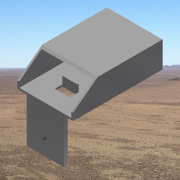
# Autodesk Inventor part: 2p1hh
Saved by Autodesk Inventor 2014 SP1 (Build 180222100, 222)
## iProperties
Company: HERA Project
Created: 2013-12-03
Part Number: 2p1hh
Material: Steel, Galvanized
Document SubType Name: Modeling
Designer: David DeBoer
Mass: 1619.54 g
Surface Area: 865.184 cm^2
Volume: 206.311 cm^3
Density: 7.85 g/cm^3
Description: end horizontal holder
Appearance: Galvanized
Author: David DeBoer
Autodesk Inventor part; units mm, degrees
ref_plane "YZ Plane" through (0, 0, 0) normal (1, 0, 0) x (0, 1, 0)
ref_plane "XZ Plane" through (0, 0, 0) normal (0, 1, 0) x (-1, 0, 0)
ref_plane "XY Plane" through (0, 0, 0) normal (0, 0, 1) x (1, 0, 0)
sketch "Sketch1" plane through (0, 0, 0) normal (0, 0, 1) x (1, 0, 0)
  line L0 (0, 0) -> (88.9, 0)
  line L1 (88.9, 0) -> (88.9, 38.1)
  line L2 (88.9, 38.1) -> (0, 38.1)
  line L3 (0, 38.1) -> (0, 0)
  line L4 (-3.048, 41.148) -> (91.948, 41.148)
  line L5 (91.948, 41.148) -> (91.948, -3.048)
  line L6 (91.948, -3.048) -> (-3.048, -3.048)
  line L7 (-3.048, -3.048) -> (-3.048, 41.148)
  dimension "d0" = 88.9
  dimension "d1" = 38.1
  dimension "d2" = 3.048
  constraints: 16 end point, 4 parallel, 2 perpendicular, 1 horizontal, 3 other
  measures "d0" distance of L0.start L0.end
  measures "d1" distance of L2.end L0.start
  measures "d2" distance between parallel lines of L4 L2
extrude "Extrusion1" add sketch "Sketch1" along normal blind 152.4
ref_plane "Work Plane1" through (-3.048, 41.148, 152.4) normal (0, 0.7986355, 0.601815) x (-1, 0, 0)
sketch "Sketch2" plane through (-3.048, 41.148, 152.4) normal (0, 0.7986355, 0.601815) x (-1, 0, 0)
  line L0 (-144.4625, 77.7875) -> (65.0875, 77.7875)
  line L1 (65.0875, 77.7875) -> (65.0875, -49.2125)
  line L2 (65.0875, -49.2125) -> (-144.4625, -49.2125)
  line L3 (-144.4625, -49.2125) -> (-144.4625, 77.7875)
  point P0 (-3.048, -96.9486)
  dimension "d8" = 127
  constraints: 8 end point, 2 parallel, 1 horizontal, 1 perpendicular
  measures "d8" distance of L2.end L0.start
extrude "Extrusion2" cut sketch "Sketch2" against normal blind 25.4
sketch "Sketch3" plane through (-3.048, -3.048, 0) normal (0, -1, 0) x (1, 0, 0)
  line L0 (94.996, 0) -> (0, 0) projected
  line L1 (0, 152.4) -> (94.996, 152.4) projected
  line L2 (15.875, 146.05) -> (79.121, 146.05)
  line L3 (79.121, 146.05) -> (79.121, 152.4)
  line L4 (79.121, 152.4) -> (15.875, 152.4)
  line L5 (15.875, 152.4) -> (15.875, 146.05)
  line L6 (47.498, 152.4) -> (47.498, 146.05) construction
  line L7 (47.498, 152.4) -> (47.498, 0) construction
  line L8 (15.875, 149.225) -> (79.121, 149.225) construction
  point P0 (3.048, 0)
  dimension "d10" = 0
  dimension "d35" = 6.35
  constraints: 14 end point, 6 midpoint, 2 parallel, 1 collinear, 1 horizontal, 1 perpendicular
  measures "d10" distance between parallel lines of L4 L1
  measures "d35" distance of L4.end L2.start
extrude "Extrusion3" add sketch "Sketch3" along normal blind 76.2
sketch "Sketch5" plane through (0, 0, 0) normal (0, 1, 0) x (1, 0, 0)
  line L0 (0, 0) -> (0, -152.4) projected
  line L1 (88.9, -152.4) -> (0, -152.4) projected
  line L2 (31.75, -110.49) -> (57.15, -110.49)
  line L3 (57.15, -110.49) -> (57.15, -107.95)
  line L4 (57.15, -107.95) -> (31.75, -107.95)
  line L5 (31.75, -107.95) -> (31.75, -110.49)
  line L6 (44.45, -152.4) -> (44.45, -68.5497) construction
  dimension "d21" = 25.4
  dimension "d22" = 2.54
  dimension "d23" = 44.45
  dimension "d24" = 31.75
  constraints: 10 end point, 3 parallel, 1 horizontal, 1 midpoint, 1 perpendicular
  measures "d21" distance of L4.end L3.end
  measures "d22" distance of L3.end L2.end
  measures "d23" distance between parallel lines of L1 L4
  measures "d24" distance between parallel lines of L5 L0
extrude "Extrusion4" add sketch "Sketch5" along normal blind 12.7
sketch "Sketch6" plane through (0, 0, 152.4) normal (0, 0, 1) x (1, 0, 0)
  line L0 (76.073, -79.248) -> (12.827, -79.248) projected
  circle A0 centre (44.45, -53.848) radius 4.2053
  dimension "d27" = 25.4
  constraints: 1 centre point
  measures "d27" distance from line of L0 A0.centre
hole "Hole2" at (44.45, -53.848, 152.4) direction (0, 0, -1) diameter 7.7978 end through all thread size "3/8-16 UNC" class "2B" standard "ANSI Unified Screw Threads"
sketch "Sketch7" plane through (0, 0, 0) normal (0, 1, 0) x (1, 0, 0)
  line L0 (57.15, -110.49) -> (31.75, -110.49) projected
  line L1 (31.75, -110.49) -> (57.15, -110.49)
  line L2 (57.15, -110.49) -> (57.15, -123.19)
  line L3 (57.15, -123.19) -> (31.75, -123.19)
  line L4 (31.75, -123.19) -> (31.75, -110.49)
  dimension "d36" = 12.7
  dimension "d37" = 25.4
  dimension "d38" = 0
  constraints: 8 end point, 2 parallel, 1 horizontal, 1 perpendicular
  measures "d36" distance of L1.end L2.end
  measures "d37" distance of L2.end L3.end
  measures "d38" distance between parallel lines of L1 L0
extrude "Extrusion5" cut sketch "Sketch7" against normal blind 25.4
sketch "Sketch9" plane through (-3.048, -3.048, 0) normal (0, -1, 0) x (1, 0, 0)
  line L0 (0, 0) -> (0, 152.4) projected
  line L1 (94.996, 0) -> (0, 0) projected
  circle A0 centre (19.05, 19.05) radius 3.175
  circle A1 centre (69.85, 19.05) radius 3.175
  circle A2 centre (44.45, 69.85) radius 3.175
  point P0 (3.048, 0)
  dimension "d59" = 6.35
  dimension "d60" = 19.05
  dimension "d61" = 19.05
  dimension "d62" = 6.35
  dimension "d63" = 50.8
  dimension "d64" = 6.35
  dimension "d65" = 50.8
  dimension "d66" = 25.4
  constraints: 3 centre point
  measures "d59" diameter of A0
  measures "d60" distance from line of L1 A0.centre
  measures "d61" distance from line of A0.centre L0
  measures "d62" diameter of A1
  measures "d63" distance of A1.centre A0.centre
  measures "d64" diameter of A2
  measures "d65" vertical distance of A0.centre A2.centre
  measures "d66" horizontal distance of A2.centre A0.centre
hole "Hole4" at (41.402, -3.048, 69.85) at (16.002, -3.048, 19.05) at (66.802, -3.048, 19.05) direction (0, 1, 0) diameter 6.35 depth 25.4 tip angle 118
body "Solid1"
